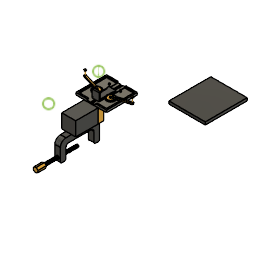
SuportTelefonMenghina (Autodesk Fusion 360 design; units mm, degrees)
part number: 2026-05-21-13-44-40-872
description: Spur Gear; Module: 1.5; Num Teeth: 18; Pressure Angle: 20.0; Backlash: 0.15 mm
part number: 2026-05-21-14-53-52-022
part number: 2026-06-04-22-19-03-842
part number: 2026-06-04-22-32-05-723
part number: 2026-06-05-00-26-46-016
part number: 2026-06-05-00-35-04-925
part number: 2026-06-05-01-32-15-649
part number: 2026-06-05-03-17-16-380
part number: 2026-06-05-03-28-47-421
part number: 2026-06-05-03-30-17-690
Autodesk Fusion 360 part; units mm, degrees
(part 1 of 5)
sketch "Sketch1" plane through (0, 0, 0) normal (0, 1, 0) x (1, 0, 0)
  line L0 (100, 100) -> (200, 100)
  line L1 (200, 100) -> (200, 0)
  line L2 (200, 0) -> (100, 0)
  line L3 (100, 0) -> (100, 100)
  line L4 (205, -5) -> (95, -5)
  line L5 (95, -5) -> (95, 105)
  line L6 (95, 105) -> (205, 105)
  line L7 (205, 105) -> (205, -5)
  dimension "d1" = 100
  dimension "d2" = 100
  dimension "d17" = -5
  constraint horizontal L0
  constraint vertical L1
  constraint horizontal L2
  constraint vertical L3
  measures "d1" distance of L0.start L0.end
  measures "d2" distance of L0.start L2.end
sketch "Base Circle" plane through (0, 0, 0) normal (0, 0, 1) x (1, 0, 0) in component "Spur Gear 18 teeth"
  circle A0 centre (0, 0) radius 11.7645
  circle A1 centre (0, 0) radius 4
extrude "Extrude1" add sketch "Base Circle" along normal blind 5 makes body 1 in component "Spur Gear 18 teeth"
sketch "Gear Tooth" plane through (0, 0, 0) normal (0, 0, 1) x (1, 0, 0) in component "Spur Gear 18 teeth"
  spline S0 degree 5 poles (12.6232, -1.2588) (12.63, -1.2595) (12.6435, -1.2606) (12.6638, -1.2618) (12.691, -1.2624) (12.725, -1.2616) (12.759, -1.2597) (12.7931, -1.2572) (12.8272, -1.2543) (12.8613, -1.2512) (12.8954, -1.2479) (12.9296, -1.2442) (12.9638, -1.2401) (12.998, -1.2355) (13.0322, -1.2304) (13.0664, -1.2248) (13.1006, -1.2188) (13.1348, -1.2124) (13.169, -1.2058) (13.2032, -1.1988) (13.2374, -1.1916) (13.2717, -1.1841) (13.3059, -1.1763) (13.3401, -1.1681) (13.3743, -1.1596) (13.4085, -1.1509) (13.4427, -1.1418) (13.4768, -1.1325) (13.511, -1.1228) (13.5452, -1.113) (13.5793, -1.1028) (13.6134, -1.0924) (13.6476, -1.0818) (13.6817, -1.0709) (13.7158, -1.0597) (13.7498, -1.0483) (13.7839, -1.0366) (13.8179, -1.0247) (13.852, -1.0125) (13.886, -1.0001) (13.9199, -0.9875) (13.9539, -0.9746) (13.9878, -0.9616) (14.0218, -0.9482) (14.0557, -0.9347) (14.0895, -0.9209) (14.1234, -0.9069) (14.1572, -0.8927) (14.191, -0.8782) (14.2248, -0.8636) (14.2585, -0.8487) (14.2922, -0.8336) (14.3259, -0.8183) (14.3596, -0.8028) (14.3932, -0.787) (14.4268, -0.7711) (14.4603, -0.755) (14.4939, -0.7386) (14.5274, -0.7221) (14.5608, -0.7053) (14.5943, -0.6884) (14.6277, -0.6712) (14.6611, -0.6538) (14.6944, -0.6363) (14.7277, -0.6185) (14.7609, -0.6006) (14.7942, -0.5824) (14.8273, -0.5641) (14.8605, -0.5456) (14.8936, -0.5269) (14.9266, -0.5079) (14.9531, -0.4927) (14.9729, -0.4811) (14.9861, -0.4734) (14.9927, -0.4695) knots 0 0 0 0 0 0 0.01428571 0.02857143 0.04285714 0.05714286 0.07142857 0.08571429 0.1 0.11428571 0.12857143 0.14285714 0.15714286 0.17142857 0.18571429 0.2 0.21428571 0.22857143 0.24285714 0.25714286 0.27142857 0.28571429 0.3 0.31428571 0.32857143 0.34285714 0.35714286 0.37142857 0.38571429 0.4 0.41428571 0.42857143 0.44285714 0.45714286 0.47142857 0.48571429 0.5 0.51428571 0.52857143 0.54285714 0.55714286 0.57142857 0.58571429 0.6 0.61428571 0.62857143 0.64285714 0.65714286 0.67142857 0.68571429 0.7 0.71428571 0.72857143 0.74285714 0.75714286 0.77142857 0.78571429 0.8 0.81428571 0.82857143 0.84285714 0.85714286 0.87142857 0.88571429 0.9 0.91428571 0.92857143 0.94285714 0.95714286 0.97142857 0.98571429 1 1 1 1 1 1
  spline S1 degree 5 poles (12.6232, 1.2588) (12.63, 1.2595) (12.6435, 1.2606) (12.6638, 1.2618) (12.691, 1.2624) (12.725, 1.2616) (12.759, 1.2597) (12.7931, 1.2572) (12.8272, 1.2543) (12.8613, 1.2512) (12.8954, 1.2479) (12.9296, 1.2442) (12.9638, 1.2401) (12.998, 1.2355) (13.0322, 1.2304) (13.0664, 1.2248) (13.1006, 1.2188) (13.1348, 1.2124) (13.169, 1.2058) (13.2032, 1.1988) (13.2374, 1.1916) (13.2717, 1.1841) (13.3059, 1.1763) (13.3401, 1.1681) (13.3743, 1.1596) (13.4085, 1.1509) (13.4427, 1.1418) (13.4768, 1.1325) (13.511, 1.1228) (13.5452, 1.113) (13.5793, 1.1028) (13.6134, 1.0924) (13.6476, 1.0818) (13.6817, 1.0709) (13.7158, 1.0597) (13.7498, 1.0483) (13.7839, 1.0366) (13.8179, 1.0247) (13.852, 1.0125) (13.886, 1.0001) (13.9199, 0.9875) (13.9539, 0.9746) (13.9878, 0.9616) (14.0218, 0.9482) (14.0557, 0.9347) (14.0895, 0.9209) (14.1234, 0.9069) (14.1572, 0.8927) (14.191, 0.8782) (14.2248, 0.8636) (14.2585, 0.8487) (14.2922, 0.8336) (14.3259, 0.8183) (14.3596, 0.8028) (14.3932, 0.787) (14.4268, 0.7711) (14.4603, 0.755) (14.4939, 0.7386) (14.5274, 0.7221) (14.5608, 0.7053) (14.5943, 0.6884) (14.6277, 0.6712) (14.6611, 0.6538) (14.6944, 0.6363) (14.7277, 0.6185) (14.7609, 0.6006) (14.7942, 0.5824) (14.8273, 0.5641) (14.8605, 0.5456) (14.8936, 0.5269) (14.9266, 0.5079) (14.9531, 0.4927) (14.9729, 0.4811) (14.9861, 0.4734) (14.9927, 0.4695) knots 0 0 0 0 0 0 0.01428571 0.02857143 0.04285714 0.05714286 0.07142857 0.08571429 0.1 0.11428571 0.12857143 0.14285714 0.15714286 0.17142857 0.18571429 0.2 0.21428571 0.22857143 0.24285714 0.25714286 0.27142857 0.28571429 0.3 0.31428571 0.32857143 0.34285714 0.35714286 0.37142857 0.38571429 0.4 0.41428571 0.42857143 0.44285714 0.45714286 0.47142857 0.48571429 0.5 0.51428571 0.52857143 0.54285714 0.55714286 0.57142857 0.58571429 0.6 0.61428571 0.62857143 0.64285714 0.65714286 0.67142857 0.68571429 0.7 0.71428571 0.72857143 0.74285714 0.75714286 0.77142857 0.78571429 0.8 0.81428571 0.82857143 0.84285714 0.85714286 0.87142857 0.88571429 0.9 0.91428571 0.92857143 0.94285714 0.95714286 0.97142857 0.98571429 1 1 1 1 1 1
  arc A0 (14.9927, -0.4695) -> (14.9927, 0.4695) centre (0, 0) ccw
  line L0 (11.6965, -1.1664) -> (12.6232, -1.2588)
  line L1 (11.6965, 1.1664) -> (12.6232, 1.2588)
  line L2 (11.6965, -1.1664) -> (11.6965, 1.1664)
  point P0 (12.7895, -1.2574)
  point P1 (12.9572, -1.2408)
  point P2 (13.1257, -1.214)
  point P3 (13.2949, -1.1787)
  point P4 (13.4645, -1.1358)
  point P5 (13.6345, -1.0858)
  point P6 (13.8046, -1.0293)
  point P7 (13.9748, -0.9665)
  point P8 (14.1451, -0.8977)
  point P9 (14.3152, -0.8231)
  point P10 (14.4851, -0.7429)
  point P11 (14.6547, -0.6571)
  point P12 (14.8239, -0.566)
  point P13 (12.7895, 1.2574)
  point P14 (12.9572, 1.2408)
  point P15 (13.1257, 1.214)
  point P16 (13.2949, 1.1787)
  point P17 (13.4645, 1.1358)
  point P18 (13.6345, 1.0858)
  point P19 (13.8046, 1.0293)
  point P20 (13.9748, 0.9665)
  point P21 (14.1451, 0.8977)
  point P22 (14.3152, 0.8231)
  point P23 (14.4851, 0.7429)
  point P24 (14.6547, 0.6571)
  point P25 (14.8239, 0.566)
extrude "Extrude2" add sketch "Gear Tooth" along normal blind 5 bodies 1 in component "Spur Gear 18 teeth"
fillet "Fillet1" radius 0.5 2 edges at (11.7064, -1.1674, 2.5) (11.7064, 1.1674, 2.5) on bodies 1 in component "Spur Gear 18 teeth"
pattern_circular "C-Pattern1" count 18 over 360 about axis through (0, 0, 0) along (0, 0, 1) of "Extrude2", "Fillet1" in component "Spur Gear 18 teeth"
sketch "Diametrial Pitch Circle" plane through (0, 0, 0) normal (0, 0, 1) x (1, 0, 0) in component "Spur Gear 18 teeth"
  circle A0 centre (0, 0) radius 13.5 construction
extrude "Extrude1'" add sketch "Sketch1" along normal blind 4 separate body contours L0 L1 L2 L3 makes body 2
extrude "Extrude2'" add sketch "Sketch1" along normal blind 8 bodies 2
sketch "Sketch2" plane through (0, 0, 0) normal (0, 1, 0) x (1, 0, 0)
  circle A0 centre (125, 40) radius 3
  circle A1 centre (175, 40) radius 3
  dimension "d22" = 6
  dimension "d23" = 6
  measures "d22" diameter of A0
  measures "d23" diameter of A1
extrude "Extrude3" add sketch "Sketch2" along normal blind 10 bodies 2
move_body "Align1" bodies 1 to x (1, 0, 0) y (0, 0, 1) z (0, -1, 0) at (125, 10, -40) in component "Spur Gear 18 teeth"
sketch "SketchCremaliera" plane through (0, 4, 0) normal (0, 1, 0) x (-1, 0, 0)
  circle A0 centre (-175, -40) radius 3
  circle A1 centre (-125, -40) radius 3
  line L0 (-100, 0) -> (-200, 0)
  line L1 (-200, 0) -> (-200, -100)
  line L2 (-200, -100) -> (-100, -100)
  line L3 (-100, -100) -> (-100, 0)
  line L4 (-150, -100) -> (-150, 0) construction
  line L5 (-150, -20) -> (-163, -20)
  line L6 (-163, -10) -> (-137, -10)
  line L7 (-137, -10) -> (-137, -70)
  line L8 (-137, -70) -> (-163, -70)
  line L9 (-163, -70) -> (-163, -10)
  line L10 (-137, -70) -> (-138.5, -70) construction
  line L11 (-138.5, -70) -> (-138.5, -10) construction
  line L12 (-138.5, -60) -> (-138.5, -60)
  line L13 (-140.375, -60) -> (-140.375, -63) construction
  line L14 (-140.375, -60) -> (-140.375, -57) construction
  line L15 (-138.5, -58.822) -> (-140.375, -59.5044)
  line L16 (-138.5, -58.822) -> (-136.5047, -58.822) construction
  line L17 (-138.5, -58.822) -> (-137, -58.276)
  line L18 (-138.5, -58.822) -> (-136.9037, -58.822) construction
  line L19 (-137, -60) -> (-137, -61.724)
  line L20 (-137, -61.724) -> (-140.375, -60.4956)
  line L21 (-137, -61.724) -> (-133.4084, -61.724) construction
  line L22 (-140.375, -60.4956) -> (-140.375, -59.5044)
  point P0 (-150, -40)
  dimension "d26" = 13
  dimension "d27" = 60
  dimension "d28" = 1.5
  dimension "d29" = 3.375
  dimension "d31" = 1.178
  dimension "d32" = 160
  dimension "d33" = 20
  dimension "d34" = 1.724
  dimension "d35" = 160
  constraint midpoint L2 L4.start
  constraint midpoint L0 L4.end
  constraint coincident L4 L5.start
  constraint perpendicular L4 L5
  constraint horizontal L6
  constraint perpendicular L6 L7
  constraint parallel L6 L8
  constraint parallel L7 L9
  constraint coincident L4 P0
  constraint horizontal L10
  constraint coincident L6 L11.end
  constraint perpendicular L6 L11
  constraint coincident L7 L19.start
  constraint perpendicular L11 L12
  constraint coincident L11 L12.start
  constraint perpendicular L12 L13
  constraint perpendicular L12 L14
  constraint horizontal L16
  constraint coincident L14 L15.end
  constraint horizontal L18
  constraint coincident L7 L17.end
  constraint perpendicular L12 L19
  constraint horizontal L21
  constraint coincident L13 L20.end
  measures "d26" distance of L5.start L5.end
  measures "d27" distance of L6.end L7.end
  measures "d28" distance of L7.end L10.end
  measures "d29" distance of L19.start L13.start
  measures "d31" distance of L12.start L15.start
  measures "d32" angle of L15 L16
  measures "d33" angle of L17 L18
  measures "d34" distance of L19.start L19.end
  measures "d35" angle of L20 L21
extrude "Extrude1''" add sketch "SketchCremaliera" along normal blind 5 separate body contours L6 L7 L8 L9 L15 L17 L20 L22 | L7 L15 L17 L19 L20 L22 makes body 3 in component "CompCremaliera"
extrude "Extrude2''" cut sketch "SketchCremaliera" along normal blind 5 contours L7 L15 L17 L19 L20 L22 bodies 3 in component "CompCremaliera"
ref_plane "WorkPlane1" through (150, 6.5, -40) normal (1, 0, 0) x (0, 0, -1)
mirror "Mirror1" about plane through (150, 6.5, -40) normal (1, 0, 0) of "Extrude2''" in component "CompCremaliera"
pattern_linear "R-Pattern1" count 11 spacing 4.712 along (0, 0, 1) of "Extrude2''", "Mirror1" in component "CompCremaliera"
copy_body "Body->Comp1" bodies 2 removing the originals makes body 4 in component "compPlaca"
sketch "SkPrindereCremaliera" plane through (0, 0, -59.5) normal (0, 0, -1) x (-1, 0, 0)
  line L0 (-163, 4) -> (-137, 4)
  line L1 (-137, 4) -> (-137, 9)
  line L2 (-137, 9) -> (-163, 9)
  line L3 (-163, 9) -> (-163, 4)
  line L4 (-150, 4) -> (-152, 4)
  line L5 (-152, 4) -> (-152, 4)
  line L6 (-152, 4) -> (-150, 4)
  line L7 (-150, 4) -> (-150, 4)
  line L8 (-150, 4) -> (-148, 4)
  line L9 (-148, 4) -> (-148, 2.5)
  line L10 (-152, 4) -> (-152, 2.5)
  line L11 (-152, 2.5) -> (-153, 2.5)
  line L12 (-153, 2.5) -> (-153, 1.5)
  line L13 (-153, 1.5) -> (-147, 1.5)
  line L14 (-147, 1.5) -> (-147, 2.5)
  line L15 (-147, 2.5) -> (-148, 2.5)
  line L16 (-147.5, 4) -> (-147.5, 3)
  line L17 (-146.5, 3) -> (-147.5, 3)
  line L18 (-146.5, 1) -> (-146.5, 3)
  line L19 (-153.5, 1) -> (-146.5, 1)
  line L20 (-153.5, 3) -> (-153.5, 1)
  line L21 (-152.5, 3) -> (-153.5, 3)
  line L22 (-152.5, 4) -> (-152.5, 3)
  line L23 (-147.5, 4) -> (-148, 4)
  line L24 (-152, 4) -> (-152.5, 4)
  line L25 (-163.7, 3.3) -> (-136.3, 3.3)
  line L26 (-136.3, 3.3) -> (-136.3, 9.7)
  line L27 (-136.3, 9.7) -> (-163.7, 9.7)
  line L28 (-163.7, 9.7) -> (-163.7, 3.3)
  dimension "d63" = 1
  dimension "d69" = 0.7
  constraint horizontal L4
  constraint horizontal L6
  constraint coincident L0 L4.end
  constraint midpoint L0 L4.start
  constraint coincident L0 L8.end
  constraint perpendicular L8 L9
  constraint perpendicular L6 L10
  constraint perpendicular L10 L11
  constraint perpendicular L11 L12
  constraint perpendicular L12 L13
  constraint perpendicular L13 L14
  constraint perpendicular L9 L15
  constraint coincident L0 L16.start
  constraint perpendicular L22 L24
  measures "d63" distance of L11.end L12.end
extrude "Extrude1'''" cut sketch "SkPrindereCremaliera" along normal mid plane 180 contours L0 L10 L22 L24 L25 | L0 L4 L6 L8 L9 L10 L25 | L9 L10 L11 L12 L13 L14 L15 L16 L17 L18 L19 L20 L21 L22 L25 | L9 L10 L11 L12 L13 L14 L15 L25 | L0 L9 L16 L23 L25 bodies 4 in component "compPlaca"
extrude "Extrude3'" add sketch "SkPrindereCremaliera" against normal blind 60 contours L0 L4 L6 L8 L9 L10 L25 | L9 L10 L11 L12 L13 L14 L15 L25 sketch seen with x (1, 0, 0) y (0, 1, 0) z (0, 0, 1) at (0, 0, -10.5) bodies 3 in component "CompCremaliera"
extrude "Extrude3''" cut sketch "SkPrindereCremaliera" along normal blind 52 contours L0 L1 L2 L3 L4 L6 L8 L23 L24 | L0 L1 L2 L3 L16 L22 L25 L26 L27 L28 bodies 4 in component "compPlaca"
sketch "SamsungFold4DeschisHusa" plane through (0, 10, 0) normal (0, 1, 0) x (-1, 0, 0)
  arc A0 (-185.4088, -33.5327) -> (-184.7313, -33.389) centre (-185.1449, -33.108) ccw
  line L0 (-185.4088, -33.5327) -> (-185.7753, -33.305)
  spline S0 degree 5 poles (-185.7753, -33.305) (-185.7811, -33.3014) (-185.7927, -33.2944) (-185.8104, -33.2844) (-185.8346, -33.272) (-185.8654, -33.2577) (-185.8968, -33.2443) (-185.9285, -33.2316) (-185.9603, -33.2191) (-185.9923, -33.2068) (-186.0245, -33.1948) (-186.0567, -33.183) (-186.0892, -33.1716) (-186.1219, -33.1607) (-186.1549, -33.1502) (-186.1881, -33.1402) (-186.2214, -33.1305) (-186.2549, -33.1211) (-186.2886, -33.112) (-186.3224, -33.1031) (-186.3563, -33.0945) (-186.3903, -33.0862) (-186.4244, -33.0781) (-186.4587, -33.0704) (-186.4932, -33.0629) (-186.5277, -33.0557) (-186.5624, -33.0488) (-186.5972, -33.0421) (-186.6321, -33.0356) (-186.6671, -33.0295) (-186.7022, -33.0235) (-186.7375, -33.0178) (-186.7728, -33.0123) (-186.8082, -33.0071) (-186.8437, -33.0021) (-186.8793, -32.9973) (-186.9151, -32.9927) (-186.9509, -32.9884) (-186.9868, -32.9844) (-187.0228, -32.9805) (-187.0588, -32.9768) (-187.095, -32.9734) (-187.1312, -32.9702) (-187.1675, -32.9672) (-187.2039, -32.9644) (-187.2404, -32.9619) (-187.277, -32.9595) (-187.3136, -32.9574) (-187.3503, -32.9554) (-187.3871, -32.9537) (-187.4239, -32.9522) (-187.4608, -32.9509) (-187.4978, -32.9497) (-187.5349, -32.9488) (-187.572, -32.9481) (-187.6091, -32.9476) (-187.6464, -32.9473) (-187.6837, -32.9472) (-187.7211, -32.9473) (-187.7585, -32.9476) (-187.796, -32.9481) (-187.8335, -32.9487) (-187.8711, -32.9496) (-187.9088, -32.9507) (-187.9465, -32.9519) (-187.9843, -32.9534) (-188.0221, -32.955) (-188.0599, -32.9568) (-188.0979, -32.9589) (-188.1358, -32.9611) (-188.1738, -32.9635) (-188.2043, -32.9655) (-188.2271, -32.9672) (-188.2424, -32.9683) (-188.25, -32.9689) knots 0 0 0 0 0 0 0.01428571 0.02857143 0.04285714 0.05714286 0.07142857 0.08571429 0.1 0.11428571 0.12857143 0.14285714 0.15714286 0.17142857 0.18571429 0.2 0.21428571 0.22857143 0.24285714 0.25714286 0.27142857 0.28571429 0.3 0.31428571 0.32857143 0.34285714 0.35714286 0.37142857 0.38571429 0.4 0.41428571 0.42857143 0.44285714 0.45714286 0.47142857 0.48571429 0.5 0.51428571 0.52857143 0.54285714 0.55714286 0.57142857 0.58571429 0.6 0.61428571 0.62857143 0.64285714 0.65714286 0.67142857 0.68571429 0.7 0.71428571 0.72857143 0.74285714 0.75714286 0.77142857 0.78571429 0.8 0.81428571 0.82857143 0.84285714 0.85714286 0.87142857 0.88571429 0.9 0.91428571 0.92857143 0.94285714 0.95714286 0.97142857 0.98571429 1 1 1 1 1 1
  arc A1 (-188.25, -32.9689) -> (-188.664, -33.8117) centre (-175, -40) ccw
  spline S1 degree 5 poles (-186.8853, -35.5647) (-186.8916, -35.5624) (-186.9043, -35.5575) (-186.923, -35.5496) (-186.9476, -35.5381) (-186.9778, -35.5224) (-187.0075, -35.5057) (-187.037, -35.4884) (-187.0663, -35.4708) (-187.0956, -35.453) (-187.1248, -35.4349) (-187.1538, -35.4166) (-187.1827, -35.3978) (-187.2113, -35.3786) (-187.2398, -35.3589) (-187.268, -35.3388) (-187.296, -35.3184) (-187.324, -35.2976) (-187.3517, -35.2765) (-187.3794, -35.2552) (-187.4069, -35.2336) (-187.4343, -35.2118) (-187.4616, -35.1897) (-187.4887, -35.1673) (-187.5156, -35.1446) (-187.5425, -35.1217) (-187.5692, -35.0985) (-187.5957, -35.075) (-187.6222, -35.0513) (-187.6485, -35.0274) (-187.6746, -35.0032) (-187.7007, -34.9789) (-187.7266, -34.9543) (-187.7524, -34.9294) (-187.7781, -34.9044) (-187.8036, -34.8791) (-187.8291, -34.8536) (-187.8544, -34.8279) (-187.8795, -34.802) (-187.9046, -34.7759) (-187.9295, -34.7496) (-187.9543, -34.723) (-187.979, -34.6963) (-188.0036, -34.6694) (-188.0281, -34.6423) (-188.0524, -34.615) (-188.0766, -34.5875) (-188.1007, -34.5598) (-188.1246, -34.532) (-188.1485, -34.5039) (-188.1722, -34.4757) (-188.1958, -34.4473) (-188.2193, -34.4187) (-188.2427, -34.3899) (-188.2659, -34.361) (-188.2891, -34.3319) (-188.3121, -34.3026) (-188.335, -34.2731) (-188.3577, -34.2435) (-188.3804, -34.2137) (-188.4029, -34.1838) (-188.4253, -34.1536) (-188.4476, -34.1233) (-188.4698, -34.0929) (-188.4919, -34.0623) (-188.5138, -34.0315) (-188.5356, -34.0006) (-188.5573, -33.9695) (-188.5789, -33.9382) (-188.6004, -33.9069) (-188.6217, -33.8753) (-188.6387, -33.8499) (-188.6514, -33.8308) (-188.6598, -33.8181) (-188.664, -33.8117) knots 0 0 0 0 0 0 0.01428571 0.02857143 0.04285714 0.05714286 0.07142857 0.08571429 0.1 0.11428571 0.12857143 0.14285714 0.15714286 0.17142857 0.18571429 0.2 0.21428571 0.22857143 0.24285714 0.25714286 0.27142857 0.28571429 0.3 0.31428571 0.32857143 0.34285714 0.35714286 0.37142857 0.38571429 0.4 0.41428571 0.42857143 0.44285714 0.45714286 0.47142857 0.48571429 0.5 0.51428571 0.52857143 0.54285714 0.55714286 0.57142857 0.58571429 0.6 0.61428571 0.62857143 0.64285714 0.65714286 0.67142857 0.68571429 0.7 0.71428571 0.72857143 0.74285714 0.75714286 0.77142857 0.78571429 0.8 0.81428571 0.82857143 0.84285714 0.85714286 0.87142857 0.88571429 0.9 0.91428571 0.92857143 0.94285714 0.95714286 0.97142857 0.98571429 1 1 1 1 1 1
  line L1 (-186.8853, -35.5647) -> (-186.4809, -35.7156)
  arc A2 (-186.1806, -36.3396) -> (-186.4809, -35.7156) centre (-186.6558, -36.1841) ccw
  arc A3 (-186.1806, -36.3396) -> (-186.4055, -37.116) centre (-175, -40) ccw
  arc A4 (-186.993, -37.4828) -> (-186.4055, -37.116) centre (-186.8903, -36.9934) ccw
  line L2 (-186.993, -37.4828) -> (-187.4153, -37.3941)
  spline S2 degree 5 poles (-187.4153, -37.3941) (-187.422, -37.3927) (-187.4353, -37.3901) (-187.4554, -37.3868) (-187.4823, -37.3833) (-187.5162, -37.3805) (-187.5502, -37.3787) (-187.5843, -37.3775) (-187.6186, -37.3767) (-187.6528, -37.3761) (-187.6871, -37.3758) (-187.7215, -37.3758) (-187.7559, -37.3762) (-187.7904, -37.3771) (-187.8249, -37.3785) (-187.8595, -37.3804) (-187.8942, -37.3827) (-187.9289, -37.3854) (-187.9636, -37.3883) (-187.9984, -37.3916) (-188.0332, -37.3951) (-188.068, -37.3989) (-188.1029, -37.403) (-188.1378, -37.4074) (-188.1727, -37.4121) (-188.2076, -37.4172) (-188.2426, -37.4226) (-188.2776, -37.4282) (-188.3126, -37.4341) (-188.3476, -37.4402) (-188.3826, -37.4466) (-188.4177, -37.4533) (-188.4527, -37.4602) (-188.4878, -37.4674) (-188.5229, -37.4749) (-188.558, -37.4826) (-188.5931, -37.4905) (-188.6282, -37.4987) (-188.6634, -37.5072) (-188.6985, -37.5158) (-188.7336, -37.5247) (-188.7688, -37.5339) (-188.8039, -37.5433) (-188.8391, -37.5529) (-188.8742, -37.5627) (-188.9094, -37.5728) (-188.9446, -37.5831) (-188.9797, -37.5936) (-189.0149, -37.6043) (-189.05, -37.6153) (-189.0851, -37.6264) (-189.1203, -37.6378) (-189.1554, -37.6494) (-189.1905, -37.6612) (-189.2257, -37.6733) (-189.2608, -37.6855) (-189.2959, -37.698) (-189.331, -37.7106) (-189.3661, -37.7235) (-189.4011, -37.7365) (-189.4362, -37.7498) (-189.4712, -37.7633) (-189.5063, -37.777) (-189.5413, -37.7909) (-189.5763, -37.8049) (-189.6113, -37.8192) (-189.6463, -37.8337) (-189.6812, -37.8484) (-189.7162, -37.8632) (-189.7511, -37.8783) (-189.786, -37.8935) (-189.8139, -37.9059) (-189.8348, -37.9152) (-189.8488, -37.9215) (-189.8557, -37.9247) knots 0 0 0 0 0 0 0.01428571 0.02857143 0.04285714 0.05714286 0.07142857 0.08571429 0.1 0.11428571 0.12857143 0.14285714 0.15714286 0.17142857 0.18571429 0.2 0.21428571 0.22857143 0.24285714 0.25714286 0.27142857 0.28571429 0.3 0.31428571 0.32857143 0.34285714 0.35714286 0.37142857 0.38571429 0.4 0.41428571 0.42857143 0.44285714 0.45714286 0.47142857 0.48571429 0.5 0.51428571 0.52857143 0.54285714 0.55714286 0.57142857 0.58571429 0.6 0.61428571 0.62857143 0.64285714 0.65714286 0.67142857 0.68571429 0.7 0.71428571 0.72857143 0.74285714 0.75714286 0.77142857 0.78571429 0.8 0.81428571 0.82857143 0.84285714 0.85714286 0.87142857 0.88571429 0.9 0.91428571 0.92857143 0.94285714 0.95714286 0.97142857 0.98571429 1 1 1 1 1 1
  arc A5 (-189.8557, -37.9247) -> (-189.9565, -38.8583) centre (-175, -40) ccw
  spline S3 degree 5 poles (-187.6854, -39.8972) (-187.6922, -39.8972) (-187.7058, -39.8969) (-187.7261, -39.8959) (-187.7532, -39.8935) (-187.7869, -39.889) (-187.8205, -39.8835) (-187.8541, -39.8774) (-187.8877, -39.8709) (-187.9213, -39.8642) (-187.9549, -39.8572) (-187.9885, -39.8498) (-188.022, -39.8421) (-188.0555, -39.8338) (-188.0889, -39.8251) (-188.1223, -39.8158) (-188.1557, -39.8062) (-188.1891, -39.7962) (-188.2224, -39.7859) (-188.2556, -39.7753) (-188.2889, -39.7645) (-188.3221, -39.7534) (-188.3553, -39.7419) (-188.3884, -39.7301) (-188.4215, -39.718) (-188.4546, -39.7057) (-188.4876, -39.693) (-188.5205, -39.68) (-188.5535, -39.6668) (-188.5864, -39.6533) (-188.6193, -39.6396) (-188.6521, -39.6256) (-188.6849, -39.6113) (-188.7176, -39.5968) (-188.7503, -39.582) (-188.7829, -39.567) (-188.8156, -39.5518) (-188.8481, -39.5363) (-188.8806, -39.5205) (-188.9131, -39.5046) (-188.9455, -39.4884) (-188.9779, -39.4719) (-189.0103, -39.4553) (-189.0426, -39.4384) (-189.0748, -39.4213) (-189.107, -39.4039) (-189.1392, -39.3864) (-189.1713, -39.3686) (-189.2033, -39.3506) (-189.2353, -39.3324) (-189.2673, -39.314) (-189.2992, -39.2954) (-189.331, -39.2766) (-189.3628, -39.2575) (-189.3945, -39.2383) (-189.4262, -39.2188) (-189.4579, -39.1992) (-189.4895, -39.1793) (-189.521, -39.1593) (-189.5525, -39.139) (-189.5839, -39.1186) (-189.6153, -39.0979) (-189.6466, -39.0771) (-189.6778, -39.0561) (-189.709, -39.0349) (-189.7402, -39.0134) (-189.7713, -38.9918) (-189.8023, -38.9701) (-189.8332, -38.9481) (-189.8641, -38.9259) (-189.895, -38.9036) (-189.9196, -38.8855) (-189.9381, -38.8719) (-189.9503, -38.8628) (-189.9565, -38.8583) knots 0 0 0 0 0 0 0.01428571 0.02857143 0.04285714 0.05714286 0.07142857 0.08571429 0.1 0.11428571 0.12857143 0.14285714 0.15714286 0.17142857 0.18571429 0.2 0.21428571 0.22857143 0.24285714 0.25714286 0.27142857 0.28571429 0.3 0.31428571 0.32857143 0.34285714 0.35714286 0.37142857 0.38571429 0.4 0.41428571 0.42857143 0.44285714 0.45714286 0.47142857 0.48571429 0.5 0.51428571 0.52857143 0.54285714 0.55714286 0.57142857 0.58571429 0.6 0.61428571 0.62857143 0.64285714 0.65714286 0.67142857 0.68571429 0.7 0.71428571 0.72857143 0.74285714 0.75714286 0.77142857 0.78571429 0.8 0.81428571 0.82857143 0.84285714 0.85714286 0.87142857 0.88571429 0.9 0.91428571 0.92857143 0.94285714 0.95714286 0.97142857 0.98571429 1 1 1 1 1 1
  line L3 (-187.6854, -39.8972) -> (-187.2539, -39.9007)
  arc A6 (-186.7582, -40.3844) -> (-187.2539, -39.9007) centre (-187.258, -40.4007) ccw
  arc A7 (-186.7582, -40.3844) -> (-186.7041, -41.1909) centre (-175, -40) ccw
  arc A8 (-187.1307, -41.7364) -> (-186.7041, -41.1909) centre (-187.2015, -41.2415) ccw
  line L4 (-187.1307, -41.7364) -> (-187.5578, -41.7976)
  spline S4 degree 5 poles (-187.5578, -41.7976) (-187.5646, -41.7985) (-187.578, -41.8006) (-187.598, -41.8044) (-187.6245, -41.8103) (-187.6573, -41.8192) (-187.6899, -41.8292) (-187.7224, -41.8398) (-187.7548, -41.8507) (-187.7872, -41.8619) (-187.8195, -41.8733) (-187.8518, -41.885) (-187.884, -41.8972) (-187.9161, -41.9098) (-187.9481, -41.923) (-187.98, -41.9366) (-188.0117, -41.9506) (-188.0434, -41.965) (-188.0751, -41.9797) (-188.1066, -41.9946) (-188.1381, -42.0098) (-188.1696, -42.0253) (-188.2009, -42.041) (-188.2322, -42.0571) (-188.2634, -42.0735) (-188.2945, -42.0902) (-188.3255, -42.1072) (-188.3564, -42.1245) (-188.3873, -42.142) (-188.4181, -42.1597) (-188.4488, -42.1777) (-188.4795, -42.196) (-188.5101, -42.2145) (-188.5406, -42.2333) (-188.571, -42.2523) (-188.6014, -42.2715) (-188.6316, -42.291) (-188.6618, -42.3107) (-188.692, -42.3306) (-188.722, -42.3508) (-188.752, -42.3712) (-188.7819, -42.3918) (-188.8117, -42.4127) (-188.8415, -42.4337) (-188.8711, -42.455) (-188.9007, -42.4765) (-188.9302, -42.4981) (-188.9597, -42.52) (-188.989, -42.5422) (-189.0183, -42.5645) (-189.0475, -42.587) (-189.0766, -42.6097) (-189.1057, -42.6326) (-189.1347, -42.6557) (-189.1635, -42.6791) (-189.1923, -42.7026) (-189.2211, -42.7263) (-189.2497, -42.7502) (-189.2783, -42.7743) (-189.3068, -42.7985) (-189.3352, -42.823) (-189.3635, -42.8476) (-189.3918, -42.8725) (-189.4199, -42.8975) (-189.448, -42.9227) (-189.476, -42.9481) (-189.5039, -42.9736) (-189.5317, -42.9994) (-189.5595, -43.0253) (-189.5872, -43.0514) (-189.6147, -43.0777) (-189.6367, -43.0988) (-189.6532, -43.1148) (-189.6642, -43.1254) (-189.6696, -43.1308) knots 0 0 0 0 0 0 0.01428571 0.02857143 0.04285714 0.05714286 0.07142857 0.08571429 0.1 0.11428571 0.12857143 0.14285714 0.15714286 0.17142857 0.18571429 0.2 0.21428571 0.22857143 0.24285714 0.25714286 0.27142857 0.28571429 0.3 0.31428571 0.32857143 0.34285714 0.35714286 0.37142857 0.38571429 0.4 0.41428571 0.42857143 0.44285714 0.45714286 0.47142857 0.48571429 0.5 0.51428571 0.52857143 0.54285714 0.55714286 0.57142857 0.58571429 0.6 0.61428571 0.62857143 0.64285714 0.65714286 0.67142857 0.68571429 0.7 0.71428571 0.72857143 0.74285714 0.75714286 0.77142857 0.78571429 0.8 0.81428571 0.82857143 0.84285714 0.85714286 0.87142857 0.88571429 0.9 0.91428571 0.92857143 0.94285714 0.95714286 0.97142857 0.98571429 1 1 1 1 1 1
  arc A9 (-189.6696, -43.1308) -> (-189.445, -44.0425) centre (-175, -40) ccw
  spline S5 degree 5 poles (-186.9556, -44.2421) (-186.962, -44.2444) (-186.9748, -44.2487) (-186.9943, -44.2547) (-187.0205, -44.2617) (-187.0537, -44.2691) (-187.0872, -44.2754) (-187.1208, -44.2812) (-187.1546, -44.2865) (-187.1885, -44.2917) (-187.2225, -44.2966) (-187.2565, -44.3012) (-187.2907, -44.3054) (-187.325, -44.3091) (-187.3594, -44.3123) (-187.394, -44.3151) (-187.4286, -44.3174) (-187.4634, -44.3194) (-187.4982, -44.3211) (-187.5331, -44.3226) (-187.568, -44.3238) (-187.603, -44.3247) (-187.6381, -44.3252) (-187.6733, -44.3255) (-187.7085, -44.3255) (-187.7438, -44.3251) (-187.7792, -44.3245) (-187.8146, -44.3236) (-187.8501, -44.3225) (-187.8856, -44.321) (-187.9212, -44.3194) (-187.9568, -44.3174) (-187.9925, -44.3153) (-188.0282, -44.3128) (-188.064, -44.3101) (-188.0998, -44.3072) (-188.1357, -44.304) (-188.1716, -44.3006) (-188.2075, -44.2969) (-188.2435, -44.293) (-188.2795, -44.2889) (-188.3156, -44.2845) (-188.3517, -44.2799) (-188.3878, -44.2751) (-188.4239, -44.27) (-188.4601, -44.2648) (-188.4963, -44.2593) (-188.5326, -44.2535) (-188.5688, -44.2476) (-188.6051, -44.2415) (-188.6415, -44.2351) (-188.6778, -44.2285) (-188.7142, -44.2217) (-188.7506, -44.2147) (-188.787, -44.2075) (-188.8234, -44.2) (-188.8599, -44.1924) (-188.8963, -44.1845) (-188.9328, -44.1765) (-188.9693, -44.1682) (-189.0058, -44.1597) (-189.0424, -44.1511) (-189.0789, -44.1422) (-189.1155, -44.1331) (-189.1521, -44.1238) (-189.1886, -44.1144) (-189.2252, -44.1047) (-189.2618, -44.0948) (-189.2985, -44.0848) (-189.3351, -44.0745) (-189.3717, -44.0641) (-189.401, -44.0556) (-189.423, -44.0491) (-189.4377, -44.0447) (-189.445, -44.0425) knots 0 0 0 0 0 0 0.01428571 0.02857143 0.04285714 0.05714286 0.07142857 0.08571429 0.1 0.11428571 0.12857143 0.14285714 0.15714286 0.17142857 0.18571429 0.2 0.21428571 0.22857143 0.24285714 0.25714286 0.27142857 0.28571429 0.3 0.31428571 0.32857143 0.34285714 0.35714286 0.37142857 0.38571429 0.4 0.41428571 0.42857143 0.44285714 0.45714286 0.47142857 0.48571429 0.5 0.51428571 0.52857143 0.54285714 0.55714286 0.57142857 0.58571429 0.6 0.61428571 0.62857143 0.64285714 0.65714286 0.67142857 0.68571429 0.7 0.71428571 0.72857143 0.74285714 0.75714286 0.77142857 0.78571429 0.8 0.81428571 0.82857143 0.84285714 0.85714286 0.87142857 0.88571429 0.9 0.91428571 0.92857143 0.94285714 0.95714286 0.97142857 0.98571429 1 1 1 1 1 1
  line L5 (-186.9556, -44.2421) -> (-186.5489, -44.0978)
  arc A10 (-185.9177, -44.3827) -> (-186.5489, -44.0978) centre (-186.3817, -44.569) ccw
  arc A11 (-185.9177, -44.3827) -> (-185.5909, -45.1221) centre (-175, -40) ccw
  arc A12 (-185.8052, -45.7806) -> (-185.5909, -45.1221) centre (-186.0411, -45.3398) ccw
  line L6 (-185.8052, -45.7806) -> (-186.1857, -45.9842)
  spline S6 degree 5 poles (-186.1857, -45.9842) (-186.1917, -45.9874) (-186.2036, -45.994) (-186.2211, -46.0043) (-186.2439, -46.019) (-186.2717, -46.0386) (-186.299, -46.0591) (-186.3259, -46.0801) (-186.3526, -46.1015) (-186.3792, -46.1231) (-186.4057, -46.1449) (-186.432, -46.1669) (-186.4581, -46.1894) (-186.484, -46.2122) (-186.5095, -46.2355) (-186.5348, -46.2592) (-186.5599, -46.2833) (-186.5848, -46.3076) (-186.6095, -46.3322) (-186.634, -46.357) (-186.6584, -46.3821) (-186.6827, -46.4074) (-186.7067, -46.4329) (-186.7306, -46.4587) (-186.7543, -46.4848) (-186.7778, -46.5111) (-186.8011, -46.5377) (-186.8243, -46.5645) (-186.8474, -46.5915) (-186.8702, -46.6187) (-186.8929, -46.6462) (-186.9155, -46.6738) (-186.9379, -46.7017) (-186.9602, -46.7297) (-186.9823, -46.758) (-187.0042, -46.7865) (-187.026, -46.8151) (-187.0476, -46.844) (-187.0691, -46.873) (-187.0905, -46.9023) (-187.1116, -46.9317) (-187.1327, -46.9613) (-187.1536, -46.991) (-187.1743, -47.021) (-187.1949, -47.0511) (-187.2154, -47.0814) (-187.2357, -47.1119) (-187.2559, -47.1426) (-187.2759, -47.1734) (-187.2958, -47.2044) (-187.3155, -47.2355) (-187.3351, -47.2668) (-187.3546, -47.2983) (-187.3739, -47.3299) (-187.3931, -47.3617) (-187.4121, -47.3937) (-187.431, -47.4258) (-187.4498, -47.458) (-187.4684, -47.4904) (-187.4868, -47.523) (-187.5052, -47.5557) (-187.5233, -47.5885) (-187.5414, -47.6215) (-187.5593, -47.6547) (-187.5771, -47.6879) (-187.5947, -47.7214) (-187.6122, -47.7549) (-187.6295, -47.7887) (-187.6467, -47.8225) (-187.6638, -47.8565) (-187.6807, -47.8906) (-187.6942, -47.918) (-187.7042, -47.9386) (-187.7108, -47.9524) (-187.7142, -47.9593) knots 0 0 0 0 0 0 0.01428571 0.02857143 0.04285714 0.05714286 0.07142857 0.08571429 0.1 0.11428571 0.12857143 0.14285714 0.15714286 0.17142857 0.18571429 0.2 0.21428571 0.22857143 0.24285714 0.25714286 0.27142857 0.28571429 0.3 0.31428571 0.32857143 0.34285714 0.35714286 0.37142857 0.38571429 0.4 0.41428571 0.42857143 0.44285714 0.45714286 0.47142857 0.48571429 0.5 0.51428571 0.52857143 0.54285714 0.55714286 0.57142857 0.58571429 0.6 0.61428571 0.62857143 0.64285714 0.65714286 0.67142857 0.68571429 0.7 0.71428571 0.72857143 0.74285714 0.75714286 0.77142857 0.78571429 0.8 0.81428571 0.82857143 0.84285714 0.85714286 0.87142857 0.88571429 0.9 0.91428571 0.92857143 0.94285714 0.95714286 0.97142857 0.98571429 1 1 1 1 1 1
  arc A13 (-187.7142, -47.9593) -> (-187.1912, -48.7392) centre (-175, -40) ccw
  spline S7 degree 5 poles (-184.7837, -48.0753) (-184.7889, -48.0796) (-184.7995, -48.0881) (-184.8157, -48.1004) (-184.838, -48.116) (-184.8666, -48.1342) (-184.8959, -48.1516) (-184.9256, -48.1685) (-184.9555, -48.1852) (-184.9856, -48.2016) (-185.0158, -48.2178) (-185.0463, -48.2338) (-185.0769, -48.2494) (-185.1079, -48.2646) (-185.1391, -48.2794) (-185.1707, -48.2938) (-185.2024, -48.3079) (-185.2344, -48.3216) (-185.2665, -48.3352) (-185.2988, -48.3485) (-185.3313, -48.3615) (-185.3639, -48.3743) (-185.3966, -48.3869) (-185.4296, -48.3992) (-185.4627, -48.4112) (-185.496, -48.4229) (-185.5294, -48.4344) (-185.563, -48.4457) (-185.5968, -48.4568) (-185.6306, -48.4676) (-185.6646, -48.4782) (-185.6988, -48.4886) (-185.733, -48.4987) (-185.7675, -48.5086) (-185.802, -48.5183) (-185.8367, -48.5278) (-185.8714, -48.5371) (-185.9064, -48.5462) (-185.9414, -48.555) (-185.9765, -48.5637) (-186.0118, -48.5721) (-186.0472, -48.5803) (-186.0826, -48.5883) (-186.1182, -48.5962) (-186.1539, -48.6038) (-186.1897, -48.6112) (-186.2256, -48.6184) (-186.2617, -48.6254) (-186.2978, -48.6323) (-186.334, -48.6389) (-186.3703, -48.6453) (-186.4067, -48.6516) (-186.4432, -48.6576) (-186.4798, -48.6635) (-186.5165, -48.6691) (-186.5533, -48.6746) (-186.5901, -48.6799) (-186.6271, -48.685) (-186.6641, -48.6899) (-186.7013, -48.6946) (-186.7385, -48.6992) (-186.7758, -48.7035) (-186.8131, -48.7077) (-186.8506, -48.7116) (-186.8881, -48.7154) (-186.9258, -48.7191) (-186.9635, -48.7225) (-187.0012, -48.7257) (-187.0391, -48.7288) (-187.077, -48.7317) (-187.115, -48.7344) (-187.1455, -48.7364) (-187.1683, -48.7378) (-187.1836, -48.7388) (-187.1912, -48.7392) knots 0 0 0 0 0 0 0.01428571 0.02857143 0.04285714 0.05714286 0.07142857 0.08571429 0.1 0.11428571 0.12857143 0.14285714 0.15714286 0.17142857 0.18571429 0.2 0.21428571 0.22857143 0.24285714 0.25714286 0.27142857 0.28571429 0.3 0.31428571 0.32857143 0.34285714 0.35714286 0.37142857 0.38571429 0.4 0.41428571 0.42857143 0.44285714 0.45714286 0.47142857 0.48571429 0.5 0.51428571 0.52857143 0.54285714 0.55714286 0.57142857 0.58571429 0.6 0.61428571 0.62857143 0.64285714 0.65714286 0.67142857 0.68571429 0.7 0.71428571 0.72857143 0.74285714 0.75714286 0.77142857 0.78571429 0.8 0.81428571 0.82857143 0.84285714 0.85714286 0.87142857 0.88571429 0.9 0.91428571 0.92857143 0.94285714 0.95714286 0.97142857 0.98571429 1 1 1 1 1 1
  line L7 (-184.7837, -48.0753) -> (-184.4509, -47.8006)
  arc A14 (-183.7603, -47.8525) -> (-184.4509, -47.8006) centre (-184.1326, -48.1862) ccw
  arc A15 (-183.7603, -47.8525) -> (-183.2004, -48.4355) centre (-175, -40) ccw
  arc A16 (-183.1765, -49.1276) -> (-183.2004, -48.4355) centre (-183.5489, -48.794) ccw
  line L8 (-183.1765, -49.1276) -> (-183.4644, -49.4491)
  spline S8 degree 5 poles (-183.4644, -49.4491) (-183.4689, -49.4541) (-183.4779, -49.4643) (-183.4908, -49.48) (-183.5072, -49.5016) (-183.5266, -49.5296) (-183.5452, -49.5581) (-183.5633, -49.5871) (-183.5811, -49.6163) (-183.5988, -49.6457) (-183.6162, -49.6753) (-183.6334, -49.705) (-183.6502, -49.735) (-183.6667, -49.7653) (-183.6827, -49.796) (-183.6984, -49.8269) (-183.7137, -49.8581) (-183.7288, -49.8894) (-183.7436, -49.921) (-183.7582, -49.9527) (-183.7725, -49.9846) (-183.7867, -50.0167) (-183.8005, -50.0489) (-183.8141, -50.0813) (-183.8275, -50.1139) (-183.8406, -50.1467) (-183.8534, -50.1797) (-183.866, -50.2128) (-183.8784, -50.246) (-183.8906, -50.2794) (-183.9026, -50.313) (-183.9143, -50.3467) (-183.9259, -50.3805) (-183.9372, -50.4145) (-183.9483, -50.4486) (-183.9592, -50.4829) (-183.9698, -50.5173) (-183.9803, -50.5518) (-183.9905, -50.5864) (-184.0006, -50.6212) (-184.0105, -50.6561) (-184.0201, -50.6911) (-184.0296, -50.7262) (-184.0388, -50.7614) (-184.0479, -50.7968) (-184.0567, -50.8323) (-184.0654, -50.8679) (-184.0739, -50.9036) (-184.0822, -50.9394) (-184.0902, -50.9753) (-184.0981, -51.0113) (-184.1058, -51.0474) (-184.1134, -51.0837) (-184.1207, -51.12) (-184.1278, -51.1564) (-184.1348, -51.193) (-184.1416, -51.2296) (-184.1482, -51.2663) (-184.1546, -51.3031) (-184.1608, -51.34) (-184.1668, -51.377) (-184.1727, -51.4141) (-184.1783, -51.4513) (-184.1838, -51.4886) (-184.1891, -51.5259) (-184.1943, -51.5634) (-184.1992, -51.6009) (-184.204, -51.6385) (-184.2086, -51.6762) (-184.213, -51.714) (-184.2173, -51.7518) (-184.2205, -51.7822) (-184.2229, -51.805) (-184.2244, -51.8202) (-184.2252, -51.8278) knots 0 0 0 0 0 0 0.01428571 0.02857143 0.04285714 0.05714286 0.07142857 0.08571429 0.1 0.11428571 0.12857143 0.14285714 0.15714286 0.17142857 0.18571429 0.2 0.21428571 0.22857143 0.24285714 0.25714286 0.27142857 0.28571429 0.3 0.31428571 0.32857143 0.34285714 0.35714286 0.37142857 0.38571429 0.4 0.41428571 0.42857143 0.44285714 0.45714286 0.47142857 0.48571429 0.5 0.51428571 0.52857143 0.54285714 0.55714286 0.57142857 0.58571429 0.6 0.61428571 0.62857143 0.64285714 0.65714286 0.67142857 0.68571429 0.7 0.71428571 0.72857143 0.74285714 0.75714286 0.77142857 0.78571429 0.8 0.81428571 0.82857143 0.84285714 0.85714286 0.87142857 0.88571429 0.9 0.91428571 0.92857143 0.94285714 0.95714286 0.97142857 0.98571429 1 1 1 1 1 1
  arc A17 (-184.2252, -51.8278) -> (-183.467, -52.3818) centre (-175, -40) ccw
  spline S9 degree 5 poles (-181.4317, -50.9345) (-181.4352, -50.9404) (-181.4422, -50.952) (-181.4532, -50.9691) (-181.4688, -50.9913) (-181.4895, -51.0183) (-181.5111, -51.0446) (-181.5332, -51.0707) (-181.5557, -51.0965) (-181.5783, -51.1223) (-181.6011, -51.1478) (-181.6243, -51.1733) (-181.6477, -51.1984) (-181.6716, -51.2233) (-181.696, -51.2479) (-181.7207, -51.2722) (-181.7457, -51.2963) (-181.771, -51.3202) (-181.7966, -51.3439) (-181.8224, -51.3674) (-181.8484, -51.3908) (-181.8746, -51.4139) (-181.9011, -51.437) (-181.9279, -51.4598) (-181.9549, -51.4824) (-181.9822, -51.5048) (-182.0097, -51.5271) (-182.0374, -51.5491) (-182.0653, -51.5711) (-182.0934, -51.5928) (-182.1218, -51.6144) (-182.1503, -51.6358) (-182.179, -51.6571) (-182.208, -51.6782) (-182.2371, -51.6991) (-182.2664, -51.7199) (-182.296, -51.7405) (-182.3257, -51.761) (-182.3555, -51.7813) (-182.3856, -51.8014) (-182.4159, -51.8214) (-182.4463, -51.8412) (-182.4769, -51.8609) (-182.5077, -51.8804) (-182.5386, -51.8998) (-182.5697, -51.919) (-182.601, -51.9381) (-182.6324, -51.957) (-182.664, -51.9757) (-182.6958, -51.9944) (-182.7277, -52.0128) (-182.7598, -52.0311) (-182.792, -52.0493) (-182.8244, -52.0673) (-182.8569, -52.0852) (-182.8896, -52.1029) (-182.9225, -52.1205) (-182.9554, -52.1379) (-182.9886, -52.1552) (-183.0219, -52.1723) (-183.0553, -52.1893) (-183.0888, -52.2062) (-183.1225, -52.2229) (-183.1564, -52.2394) (-183.1904, -52.2558) (-183.2245, -52.2721) (-183.2587, -52.2882) (-183.2931, -52.3042) (-183.3276, -52.32) (-183.3623, -52.3357) (-183.397, -52.3512) (-183.425, -52.3635) (-183.446, -52.3727) (-183.46, -52.3788) (-183.467, -52.3818) knots 0 0 0 0 0 0 0.01428571 0.02857143 0.04285714 0.05714286 0.07142857 0.08571429 0.1 0.11428571 0.12857143 0.14285714 0.15714286 0.17142857 0.18571429 0.2 0.21428571 0.22857143 0.24285714 0.25714286 0.27142857 0.28571429 0.3 0.31428571 0.32857143 0.34285714 0.35714286 0.37142857 0.38571429 0.4 0.41428571 0.42857143 0.44285714 0.45714286 0.47142857 0.48571429 0.5 0.51428571 0.52857143 0.54285714 0.55714286 0.57142857 0.58571429 0.6 0.61428571 0.62857143 0.64285714 0.65714286 0.67142857 0.68571429 0.7 0.71428571 0.72857143 0.74285714 0.75714286 0.77142857 0.78571429 0.8 0.81428571 0.82857143 0.84285714 0.85714286 0.87142857 0.88571429 0.9 0.91428571 0.92857143 0.94285714 0.95714286 0.97142857 0.98571429 1 1 1 1 1 1
  line L9 (-181.4317, -50.9345) -> (-181.2129, -50.5625)
  arc A18 (-180.5462, -50.3751) -> (-181.2129, -50.5625) centre (-180.782, -50.816) ccw
  arc A19 (-180.5462, -50.3751) -> (-179.8207, -50.7315) centre (-175, -40) ccw
  arc A20 (-179.5615, -51.3737) -> (-179.8207, -50.7315) centre (-180.0256, -51.1875) ccw
  line L10 (-179.5615, -51.3737) -> (-179.7222, -51.7742)
  spline S10 degree 5 poles (-179.7222, -51.7742) (-179.7247, -51.7805) (-179.7296, -51.7932) (-179.7364, -51.8124) (-179.7444, -51.8383) (-179.7531, -51.8711) (-179.7608, -51.9043) (-179.7679, -51.9378) (-179.7746, -51.9713) (-179.7812, -52.005) (-179.7874, -52.0387) (-179.7934, -52.0725) (-179.799, -52.1065) (-179.8041, -52.1406) (-179.8087, -52.1749) (-179.8128, -52.2093) (-179.8166, -52.2438) (-179.82, -52.2785) (-179.8231, -52.3132) (-179.826, -52.348) (-179.8286, -52.3828) (-179.8309, -52.4178) (-179.8329, -52.4528) (-179.8346, -52.488) (-179.8359, -52.5232) (-179.837, -52.5585) (-179.8378, -52.5938) (-179.8384, -52.6292) (-179.8387, -52.6647) (-179.8387, -52.7003) (-179.8384, -52.7359) (-179.838, -52.7716) (-179.8372, -52.8073) (-179.8362, -52.8431) (-179.835, -52.879) (-179.8335, -52.9149) (-179.8318, -52.9508) (-179.8298, -52.9869) (-179.8276, -53.0229) (-179.8251, -53.059) (-179.8225, -53.0952) (-179.8196, -53.1314) (-179.8164, -53.1676) (-179.8131, -53.2039) (-179.8095, -53.2402) (-179.8057, -53.2766) (-179.8017, -53.313) (-179.7974, -53.3495) (-179.7929, -53.3859) (-179.7883, -53.4224) (-179.7834, -53.459) (-179.7782, -53.4956) (-179.7729, -53.5322) (-179.7674, -53.5688) (-179.7616, -53.6055) (-179.7557, -53.6422) (-179.7495, -53.679) (-179.7431, -53.7157) (-179.7366, -53.7525) (-179.7298, -53.7893) (-179.7228, -53.8261) (-179.7156, -53.863) (-179.7082, -53.8999) (-179.7007, -53.9368) (-179.6929, -53.9737) (-179.6849, -54.0106) (-179.6767, -54.0476) (-179.6683, -54.0846) (-179.6598, -54.1215) (-179.651, -54.1586) (-179.642, -54.1956) (-179.6347, -54.2252) (-179.6291, -54.2474) (-179.6254, -54.2623) (-179.6235, -54.2697) knots 0 0 0 0 0 0 0.01428571 0.02857143 0.04285714 0.05714286 0.07142857 0.08571429 0.1 0.11428571 0.12857143 0.14285714 0.15714286 0.17142857 0.18571429 0.2 0.21428571 0.22857143 0.24285714 0.25714286 0.27142857 0.28571429 0.3 0.31428571 0.32857143 0.34285714 0.35714286 0.37142857 0.38571429 0.4 0.41428571 0.42857143 0.44285714 0.45714286 0.47142857 0.48571429 0.5 0.51428571 0.52857143 0.54285714 0.55714286 0.57142857 0.58571429 0.6 0.61428571 0.62857143 0.64285714 0.65714286 0.67142857 0.68571429 0.7 0.71428571 0.72857143 0.74285714 0.75714286 0.77142857 0.78571429 0.8 0.81428571 0.82857143 0.84285714 0.85714286 0.87142857 0.88571429 0.9 0.91428571 0.92857143 0.94285714 0.95714286 0.97142857 0.98571429 1 1 1 1 1 1
  arc A21 (-179.6235, -54.2697) -> (-178.7216, -54.531) centre (-175, -40) ccw
  spline S11 degree 5 poles (-177.304, -52.4749) (-177.3053, -52.4815) (-177.3079, -52.4949) (-177.3124, -52.5147) (-177.3195, -52.5409) (-177.3297, -52.5733) (-177.3409, -52.6055) (-177.3528, -52.6375) (-177.3651, -52.6695) (-177.3775, -52.7014) (-177.3903, -52.7333) (-177.4033, -52.7651) (-177.4167, -52.7967) (-177.4307, -52.8283) (-177.4451, -52.8597) (-177.46, -52.891) (-177.4753, -52.9222) (-177.491, -52.9533) (-177.5069, -52.9843) (-177.5231, -53.0152) (-177.5395, -53.0461) (-177.5563, -53.0769) (-177.5733, -53.1076) (-177.5906, -53.1381) (-177.6083, -53.1686) (-177.6262, -53.199) (-177.6445, -53.2293) (-177.6629, -53.2596) (-177.6817, -53.2897) (-177.7007, -53.3198) (-177.7199, -53.3498) (-177.7394, -53.3797) (-177.7591, -53.4095) (-177.7791, -53.4392) (-177.7993, -53.4688) (-177.8198, -53.4984) (-177.8405, -53.5278) (-177.8614, -53.5572) (-177.8825, -53.5865) (-177.9039, -53.6157) (-177.9255, -53.6448) (-177.9473, -53.6739) (-177.9693, -53.7028) (-177.9915, -53.7317) (-178.014, -53.7605) (-178.0367, -53.7892) (-178.0595, -53.8178) (-178.0826, -53.8463) (-178.1059, -53.8748) (-178.1294, -53.9031) (-178.153, -53.9314) (-178.1769, -53.9596) (-178.201, -53.9877) (-178.2253, -54.0157) (-178.2497, -54.0436) (-178.2744, -54.0714) (-178.2992, -54.0992) (-178.3243, -54.1268) (-178.3495, -54.1544) (-178.3749, -54.1819) (-178.4005, -54.2093) (-178.4263, -54.2366) (-178.4522, -54.2638) (-178.4784, -54.2909) (-178.5047, -54.318) (-178.5312, -54.3449) (-178.5578, -54.3718) (-178.5847, -54.3985) (-178.6117, -54.4252) (-178.6389, -54.4518) (-178.6663, -54.4783) (-178.6883, -54.4994) (-178.7049, -54.5152) (-178.716, -54.5257) (-178.7216, -54.531) knots 0 0 0 0 0 0 0.01428571 0.02857143 0.04285714 0.05714286 0.07142857 0.08571429 0.1 0.11428571 0.12857143 0.14285714 0.15714286 0.17142857 0.18571429 0.2 0.21428571 0.22857143 0.24285714 0.25714286 0.27142857 0.28571429 0.3 0.31428571 0.32857143 0.34285714 0.35714286 0.37142857 0.38571429 0.4 0.41428571 0.42857143 0.44285714 0.45714286 0.47142857 0.48571429 0.5 0.51428571 0.52857143 0.54285714 0.55714286 0.57142857 0.58571429 0.6 0.61428571 0.62857143 0.64285714 0.65714286 0.67142857 0.68571429 0.7 0.71428571 0.72857143 0.74285714 0.75714286 0.77142857 0.78571429 0.8 0.81428571 0.82857143 0.84285714 0.85714286 0.87142857 0.88571429 0.9 0.91428571 0.92857143 0.94285714 0.95714286 0.97142857 0.98571429 1 1 1 1 1 1
  line L11 (-177.304, -52.4749) -> (-177.2256, -52.0505)
  arc A22 (-176.6633, -51.6463) -> (-177.2256, -52.0505) centre (-176.734, -52.1413) ccw
  arc A23 (-176.6633, -51.6463) -> (-175.8596, -51.7331) centre (-175, -40) ccw
  arc A24 (-175.3964, -52.2479) -> (-175.8596, -51.7331) centre (-175.8962, -52.2317) ccw
  line L12 (-175.3964, -52.2479) -> (-175.4104, -52.6792)
  spline S12 degree 5 poles (-175.4104, -52.6792) (-175.4106, -52.686) (-175.4109, -52.6996) (-175.4107, -52.7199) (-175.4094, -52.747) (-175.4063, -52.7809) (-175.4022, -52.8147) (-175.3974, -52.8485) (-175.3923, -52.8824) (-175.3869, -52.9162) (-175.3813, -52.9501) (-175.3753, -52.9839) (-175.3689, -53.0177) (-175.362, -53.0515) (-175.3546, -53.0853) (-175.3467, -53.1191) (-175.3385, -53.1528) (-175.3298, -53.1865) (-175.3209, -53.2202) (-175.3117, -53.2539) (-175.3022, -53.2875) (-175.2924, -53.3212) (-175.2823, -53.3548) (-175.2719, -53.3884) (-175.2611, -53.4219) (-175.2501, -53.4554) (-175.2387, -53.489) (-175.2271, -53.5224) (-175.2153, -53.5559) (-175.2031, -53.5893) (-175.1907, -53.6227) (-175.1781, -53.656) (-175.1651, -53.6894) (-175.152, -53.7227) (-175.1385, -53.7559) (-175.1249, -53.7892) (-175.1109, -53.8224) (-175.0968, -53.8555) (-175.0823, -53.8887) (-175.0677, -53.9218) (-175.0528, -53.9548) (-175.0377, -53.9879) (-175.0224, -54.0208) (-175.0068, -54.0538) (-174.991, -54.0867) (-174.975, -54.1196) (-174.9588, -54.1524) (-174.9423, -54.1852) (-174.9256, -54.2179) (-174.9087, -54.2507) (-174.8916, -54.2833) (-174.8743, -54.316) (-174.8568, -54.3485) (-174.8391, -54.3811) (-174.8211, -54.4136) (-174.803, -54.446) (-174.7846, -54.4784) (-174.7661, -54.5108) (-174.7473, -54.5431) (-174.7283, -54.5754) (-174.7092, -54.6076) (-174.6898, -54.6398) (-174.6703, -54.6719) (-174.6505, -54.704) (-174.6306, -54.736) (-174.6104, -54.768) (-174.5901, -54.7999) (-174.5696, -54.8318) (-174.5489, -54.8636) (-174.528, -54.8954) (-174.5069, -54.9271) (-174.4899, -54.9525) (-174.477, -54.9715) (-174.4684, -54.9841) (-174.4641, -54.9904) knots 0 0 0 0 0 0 0.01428571 0.02857143 0.04285714 0.05714286 0.07142857 0.08571429 0.1 0.11428571 0.12857143 0.14285714 0.15714286 0.17142857 0.18571429 0.2 0.21428571 0.22857143 0.24285714 0.25714286 0.27142857 0.28571429 0.3 0.31428571 0.32857143 0.34285714 0.35714286 0.37142857 0.38571429 0.4 0.41428571 0.42857143 0.44285714 0.45714286 0.47142857 0.48571429 0.5 0.51428571 0.52857143 0.54285714 0.55714286 0.57142857 0.58571429 0.6 0.61428571 0.62857143 0.64285714 0.65714286 0.67142857 0.68571429 0.7 0.71428571 0.72857143 0.74285714 0.75714286 0.77142857 0.78571429 0.8 0.81428571 0.82857143 0.84285714 0.85714286 0.87142857 0.88571429 0.9 0.91428571 0.92857143 0.94285714 0.95714286 0.97142857 0.98571429 1 1 1 1 1 1
  arc A25 (-174.4641, -54.9904) -> (-173.5272, -54.9275) centre (-175, -40) ccw